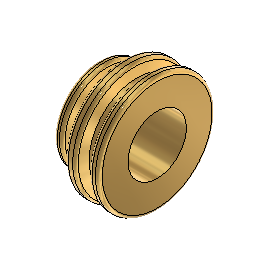
DoublePulley v3 (Autodesk Fusion 360 design; units mm, degrees)
description: Pulley
Autodesk Fusion 360 part; units mm, degrees
sketch "Sketch2" plane through (0, 0, 0) normal (0, 0, 1) x (1, 0, 0)
  line L0 (-4.9843, -7.493) -> (-5.7409, -9.8217)
  line L1 (-4.9843, -7.493) -> (-3.6995, -7.493)
  line L2 (-3.6995, -7.493) -> (-2.0076, -12.7)
  line L3 (0.7769, -10.414) -> (0.0341, -12.7)
  line L4 (0.7769, -10.414) -> (2.4231, -10.414)
  line L5 (2.4231, -10.414) -> (3.1659, -12.7)
  circle A0 centre (1.6, -12.2784) radius 1.359 construction
  line L6 (3.1659, -12.7) -> (5.1858, -12.7)
  line L7 (-2.0076, -12.7) -> (0.0341, -12.7)
  circle A1 centre (-4.3419, -8.7519) radius 1 construction
  line L8 (-7.5142, -9.8217) -> (-7.5142, -6.35)
  line L9 (-7.5142, 0) -> (5, 0)
  line L10 (-7.5142, -6.35) -> (5.1858, -6.35)
  line L11 (5.1858, -12.7) -> (5.1858, -6.35)
  line L12 (-5.7409, -9.8217) -> (-7.5142, -9.8217)
  dimension "d142_1_1_1" = 12.7
  dimension "d145_1_1_1" = 108
  dimension "d146_1_1_1" = 108
  dimension "d147_1_1_1" = 1.6
  dimension "d150_1_1_1" = 10.414
  dimension "d152_1_1_1" = 12.2784
  dimension "d158_1_1_1" = 12.7
  dimension "d159_1_1_1" = 6.35
  dimension "d161_1_1_1" = 108
  dimension "d162_1_1_1" = 7.493
  dimension "d165_1_1_1" = 108
  dimension "d166_1_1_1" = 2
  dimension "d167_1_1_1" = 7.5142
  dimension "d169_1_1_1" = 9.8217
  dimension "d64_1_1" = 1.6462
  dimension "d65_1_1" = 2.5299
  dimension "d66_1_1" = 2.0418
  constraint perpendicular L10 L11
  constraint tangent L3 A0
  constraint tangent L5 A0
  constraint horizontal L7
  constraint horizontal L6
  constraint parallel L9 L10
  constraint horizontal L1
  constraint vertical L8
  constraint horizontal L12
  constraint tangent L2 A1
  constraint tangent L0 A1
  constraint collinear L6 L7
  constraint horizontal L4
  measures "d142_1_1_1" distance of origin L6
  measures "d145_1_1_1" angle of L3 L4
  measures "d146_1_1_1" angle of L4 L5
  measures "d147_1_1_1" horizontal distance of origin A0.centre
  measures "d150_1_1_1" distance of origin L4
  measures "d152_1_1_1" vertical distance of origin A0.centre
  measures "d158_1_1_1" distance of L10.end L8.end
  measures "d159_1_1_1" distance of origin L10
  measures "d161_1_1_1" angle of L2 L7
  measures "d162_1_1_1" distance of origin L1
  measures "d165_1_1_1" angle of L0 L1
  measures "d166_1_1_1" diameter of A1
  measures "d167_1_1_1" horizontal distance of origin L8.end
  measures "d169_1_1_1" distance of origin L12
  measures "d64_1_1" distance of L3.start L4.end
  measures "d65_1_1" distance of L0.start L8
  measures "d66_1_1" distance of L3.end L2.end
revolve "Revolve2" add sketch "Sketch2" angle 360 about axis through (-7.5142, 0, 0) along (1, 0, 0)
fillet "Fillet1" radius 0.75 6 edges at (-7.5142, -3.5517, -9.1571) (-5.7409, -3.5517, -9.1571) (-2.0076, -4.5925, -11.8406) (0.0341, -4.5925, -11.8406) (3.1659, -4.5925, -11.8406) (5.1858, -4.5925, -11.8406)
equation "d116_1 = 0.0000 in"
equation "d117_1 = 0.0000 in"
equation "d118_1 = 0.0000 in"
equation "d119_1 = 0.000 deg"
equation "d128_1 = 0.0000 in"
equation "d129_1 = 0.0000 in"
equation "d130_1 = 0.0000 in"
equation "d131_1 = 0.000 deg"
